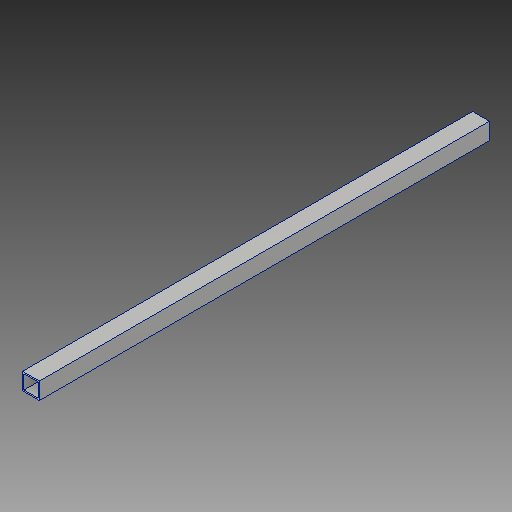
# Autodesk Inventor part: TelescopeInner
Saved by Autodesk Inventor 2018 (Build 220112000, 112)
## iProperties
Created: 2020-01-18
Part Number: TelescopeInner
Material: Aluminum 6061
Document SubType Name: Modeling
Designer: Cooper
Density: 2.7 g/cm^3
Appearance: Aluminum - Flat
Mass: 152.092 g
Surface Area: 711.894 cm^2
Volume: 56.3305 cm^3
Author: Cooper
Autodesk Inventor part; units mm, degrees
ref_plane "YZ Plane" through (0, 0, 0) normal (1, 0, 0) x (0, 1, 0)
ref_plane "XZ Plane" through (0, 0, 0) normal (0, 1, 0) x (-1, 0, 0)
ref_plane "XY Plane" through (0, 0, 0) normal (0, 0, 1) x (1, 0, 0)
sketch "Sketch1" plane through (0, 0, 0) normal (0, 0, 1) x (1, 0, 0)
  line L0 (0, 0) -> (19.05, 0)
  line L1 (19.05, 0) -> (19.05, 19.05)
  line L2 (19.05, 19.05) -> (0, 19.05)
  line L3 (0, 19.05) -> (0, 0)
  line L4 (1.5875, 17.4625) -> (17.4625, 17.4625)
  line L5 (17.4625, 17.4625) -> (17.4625, 1.5875)
  line L6 (17.4625, 1.5875) -> (1.5875, 1.5875)
  line L7 (1.5875, 1.5875) -> (1.5875, 17.4625)
  dimension "d0" = 19.05
  dimension "d1" = 19.05
  dimension "d2" = 1.5875
  constraints: 16 end point, 4 parallel, 2 perpendicular, 1 horizontal, 3 other
  measures "d0" distance of L2.end L0.start
  measures "d1" distance of L0.start L0.end
  measures "d2" distance between parallel lines of L2 L4
extrude "Extrusion1" add sketch "Sketch1" along normal blind 508
body "Solid1"
